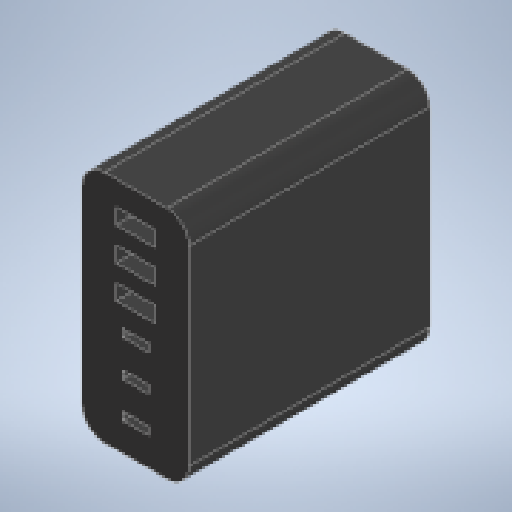
# Autodesk Inventor part: PowerUSB
Saved by Autodesk Inventor 2025.2 (Build 292293000, 293)
## iProperties
Created: 2025-08-10
Part Number: PowerUSB
Material: Generic
Document SubType Name: Modeling
Designer: hofma
Density: 1 g/cm^3
Appearance: Default
Author: hofma
Autodesk Inventor part; units mm, degrees
ref_plane "YZ Plane" through (0, 0, 0) normal (1, 0, 0) x (0, 1, 0)
ref_plane "XZ Plane" through (0, 0, 0) normal (0, 1, 0) x (-1, 0, 0)
ref_plane "XY Plane" through (0, 0, 0) normal (0, 0, 1) x (1, 0, 0)
sketch "Sketch1" plane through (0, 0, 0) normal (0, 0, 1) x (1, 0, 0)
  line L0 (-17, 37.5) -> (17, 37.5)
  line L1 (17, 37.5) -> (17, -37.5)
  line L2 (17, -37.5) -> (-17, -37.5)
  line L3 (-17, -37.5) -> (-17, 37.5)
  line L4 (-17, 37.5) -> (17, -37.5) construction
  line L5 (17, 37.5) -> (-17, -37.5) construction
  point P0 (0, 0)
  dimension "d0" = 34
  dimension "d1" = 75
  constraints: 12 end point, 2 midpoint, 2 parallel, 1 horizontal, 1 perpendicular
  measures "d0" distance of L1.end L2.end
  measures "d1" distance of L0.end L1.end
extrude "Extrusion1" add sketch "Sketch1" along normal mid plane 77
fillet "Fillet1" radius 7 4 edges at (17, 37.5, 0) (-17, 37.5, 0) (17, -37.5, 0) (-17, -37.5, 0)
sketch "Sketch2" plane through (0, 0, -38.5) normal (0, 0, -1) x (-1, 0, 0)
  circle A0 centre (0, 4.15) radius 4.1
  circle A1 centre (0, -4.15) radius 4.1
  line L0 (0, 0) -> (24.0198, 0) construction
  line L1 (-4.1, 4.15) -> (-4.1, -4.15)
  line L2 (4.1, 4.15) -> (4.1, -4.15)
  dimension "d5" = 8.2
  dimension "d6" = 16.5
  constraints: 6 end point, 4 point on circle, 4 tangent, 2 centre point, 1 equal radius, 1 horizontal, 1 vertical alignment, 1 other
  measures "d5" diameter of A0
extrude "Extrusion2" cut sketch "Sketch2" against normal blind 15
sketch "Sketch3" plane through (0, 0, -23.5) normal (0, 0, -1) x (-1, 0, 0)
  circle A0 centre (0, 4.15) radius 1
  circle A1 centre (0, -4.15) radius 1
  arc A2 (4.1, 4.15) -> (-4.1, 4.15) centre (0, 4.15) ccw projected
  arc A3 (-4.1, -4.15) -> (4.1, -4.15) centre (0, -4.15) ccw projected
  point P0 (0, 0)
  dimension "d9" = 2
  constraints: 2 centre point, 2 concentric, 1 equal radius
  measures "d9" diameter of A0
extrude "Extrusion3" add sketch "Sketch3" along normal blind 15
fillet "Fillet2" radius 1 2 edges at (1, 4.15, -38.5) (1, -4.15, -38.5)
sketch "Sketch4" plane through (0, 0, 38.5) normal (0, 0, 1) x (1, 0, 0)
  line L0 (-6.25, 29.7073) -> (6.25, 29.7073)
  line L1 (6.25, 29.7073) -> (6.25, 24.7073)
  line L2 (6.25, 24.7073) -> (-6.25, 24.7073)
  line L3 (-6.25, 24.7073) -> (-6.25, 29.7073)
  line L4 (-6.25, 29.7073) -> (6.25, 24.7073) construction
  line L5 (6.25, 29.7073) -> (-6.25, 24.7073) construction
  line L6 (-6.25, 19.2073) -> (6.25, 19.2073)
  line L7 (6.25, 19.2073) -> (6.25, 14.2073)
  line L8 (6.25, 14.2073) -> (-6.25, 14.2073)
  line L9 (-6.25, 14.2073) -> (-6.25, 19.2073)
  line L10 (-6.25, 19.2073) -> (6.25, 14.2073) construction
  line L11 (6.25, 19.2073) -> (-6.25, 14.2073) construction
  line L12 (-6.25, 8.7073) -> (6.25, 8.7073)
  line L13 (6.25, 8.7073) -> (6.25, 3.7073)
  line L14 (6.25, 3.7073) -> (-6.25, 3.7073)
  line L15 (-6.25, 3.7073) -> (-6.25, 8.7073)
  line L16 (-6.25, 8.7073) -> (6.25, 3.7073) construction
  line L17 (6.25, 8.7073) -> (-6.25, 3.7073) construction
  line L18 (-4.1, -2.8572) -> (4.1, -2.8572)
  line L19 (4.1, -2.8572) -> (4.1, -5.3572)
  line L20 (4.1, -5.3572) -> (-4.1, -5.3572)
  line L21 (-4.1, -5.3572) -> (-4.1, -2.8572)
  line L22 (-4.1, -2.8572) -> (4.1, -5.3572) construction
  line L23 (4.1, -2.8572) -> (-4.1, -5.3572) construction
  line L24 (-4.1, -14.3572) -> (4.1, -14.3572)
  line L25 (4.1, -14.3572) -> (4.1, -16.8572)
  line L26 (4.1, -16.8572) -> (-4.1, -16.8572)
  line L27 (-4.1, -16.8572) -> (-4.1, -14.3572)
  line L28 (-4.1, -14.3572) -> (4.1, -16.8572) construction
  line L29 (4.1, -14.3572) -> (-4.1, -16.8572) construction
  line L30 (-4.1, -25.8572) -> (4.1, -25.8572)
  line L31 (4.1, -25.8572) -> (4.1, -28.3572)
  line L32 (4.1, -28.3572) -> (-4.1, -28.3572)
  line L33 (-4.1, -28.3572) -> (-4.1, -25.8572)
  line L34 (-4.1, -25.8572) -> (4.1, -28.3572) construction
  line L35 (4.1, -25.8572) -> (-4.1, -28.3572) construction
  point P0 (0, 0)
  point P1 (0, 27.2073)
  point P2 (0, 16.7073)
  point P3 (0, 6.2073)
  point P4 (0, -4.1072)
  point P5 (0, -15.6072)
  point P6 (0, -27.1072)
  dimension "d5" = 8.2
  dimension "d6" = 16.5
  dimension "d14" = 12.5
  dimension "d15" = 5
  dimension "d16" = 5.5
  dimension "d17" = 5.5
  dimension "d18" = 8.2
  dimension "d19" = 2.5
  dimension "d20" = 9
  dimension "d21" = 9
  constraints: 72 end point, 12 midpoint, 12 parallel, 8 equal length, 6 horizontal, 6 perpendicular, 6 vertical alignment
  measures "d14" distance of L0.start L0.end
  measures "d15" distance of L0.end L1.end
  measures "d16" distance between parallel lines of L6 L2
  measures "d17" distance between parallel lines of L12 L8
  measures "d18" distance of L31.end L32.end
  measures "d19" distance of L18.end L19.end
  measures "d20" distance between parallel lines of L24 L20
  measures "d21" distance between parallel lines of L30 L26
extrude "Extrusion4" cut sketch "Sketch4" against normal blind 10
equation "\"d17\" = d16"
equation "\"d21\" = d20"
body "Solid1"
